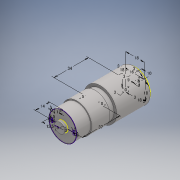
# Autodesk Inventor part: モーター100：1
Saved by Autodesk Inventor 2018 (Build 220112000, 112)
## iProperties
Part Number: モーター100：1
Material: 一般
Document SubType Name: Modeling
Designer: eieio
Density: 1 g/cm^3
Appearance: 溶接 - 軟鋼
Author: eieio
Autodesk Inventor part; units mm, degrees
ref_plane "YZ Plane" through (0, 0, 0) normal (1, 0, 0) x (0, 1, 0)
ref_plane "XZ Plane" through (0, 0, 0) normal (0, 1, 0) x (-1, 0, 0)
ref_plane "XY Plane" through (0, 0, 0) normal (0, 0, 1) x (1, 0, 0)
sketch "スケッチ1" plane through (0, 0, 0) normal (0, 0, 1) x (1, 0, 0)
  line L0 (0, 0) -> (-16, 0)
  line L1 (-16, 0) -> (-16, 34)
  line L2 (-16, 34) -> (0, 34)
  line L3 (0, 34) -> (0, 0)
  line L4 (0, 34) -> (-10, 34)
  line L5 (-10, 34) -> (-10, 37)
  line L6 (-10, 37) -> (0, 37)
  line L7 (0, 37) -> (0, 34)
  line L8 (0, 37) -> (-5, 37)
  line L9 (-5, 34) -> (0, 34)
  line L10 (0, 34) -> (0, 37)
  line L11 (-3, 37) -> (-3, 34)
  line L12 (-13.5, 0) -> (0, 0)
  line L13 (0, 0) -> (0, -37)
  line L14 (0, -37) -> (-13.5, -37)
  line L15 (-13.5, -37) -> (-13.5, 0)
  line L16 (-13.5, 0) -> (-14.5, 0)
  line L17 (-13.5, -23) -> (-13.5, 0)
  line L18 (-13.5, -5) -> (-14.5, -5)
  line L19 (-14.5, -5) -> (-14.5, -23)
  line L20 (-14.5, -23) -> (-13.5, -23)
  line L21 (-13.5, -23) -> (-13.5, -5)
  line L22 (0, -37) -> (-5, -37)
  line L23 (-5, -37) -> (-5, -40)
  line L24 (-5, -40) -> (0, -40)
  line L25 (0, -40) -> (0, -37)
  dimension "d0" = 16
  dimension "d1" = 34
  dimension "d2" = 10
  dimension "d4" = 3
  dimension "d5" = 3
  dimension "d6" = 13.5
  dimension "d7" = 0
  dimension "d10" = 37
  dimension "d11" = 5
  dimension "d12" = 14
  dimension "d13" = 1
  dimension "d14" = 3
  dimension "d15" = 5
  constraints: 52 end point, 11 parallel, 7 horizontal, 6 perpendicular, 4 point on line, 1 midpoint
  measures "d0" distance between parallel lines of L3 L1
  measures "d1" distance between parallel lines of L0 L2
  measures "d2" distance between parallel lines of L7 L5
  measures "d4" distance between parallel lines of L7 L11
  measures "d5" distance between parallel lines of L2 L6
  measures "d6" distance between parallel lines of L13 L15
  measures "d7" distance between parallel lines of L3 L13
  measures "d10" distance between parallel lines of L12 L14
  measures "d11" distance from line of L16.end L18
  measures "d12" distance from line of L20.end L14
  measures "d13" distance between parallel lines of L17 L19
  measures "d14" distance between parallel lines of L22 L24
  measures "d15" distance between parallel lines of L25 L23
revolve "回転1" add sketch "スケッチ1" angle 360 about axis through (0, 34, 0) along (0, -1, 0) contours L13 L14 L15 L0 | L0 L1 L2 L3 | L25 L24 L23 L14 | L15 L20 L19 L18 | L2 L5 L6 L11
chamfer "面取り1" distance 1 angle 45 1 edges at (16, 34, 0)
sketch "スケッチ2" plane through (0, -37, 0) normal (0, -1, 0) x (1, 0, 0)
  circle A0 centre (0, 0) radius 5 projected
  circle A1 centre (0, 0) radius 13.4
  circle A2 centre (0, 0) radius 13.5
  circle A3 centre (0, 0) radius 13.5 projected
  line L0 (-9.9, -2) -> (-11.4, -2)
  line L1 (-11.4, -2) -> (-11.4, 2)
  line L2 (-11.4, 2) -> (-9.9, 2)
  line L3 (-9.9, 2) -> (-9.9, -2)
  line L4 (-9.9, -2) -> (-11.4, 2) construction
  line L5 (-11.4, -2) -> (-9.9, 2) construction
  line L6 (11.4, -2) -> (9.9, -2)
  line L7 (9.9, -2) -> (9.9, 2)
  line L8 (9.9, 2) -> (11.4, 2)
  line L9 (11.4, 2) -> (11.4, -2)
  line L10 (11.4, -2) -> (9.9, 2) construction
  line L11 (9.9, -2) -> (11.4, 2) construction
  line L12 (-13.4, 0) -> (0, 0)
  line L13 (0, 0) -> (13.4, 0)
  point P0 (-10.65, 0)
  point P1 (10.65, 0)
  dimension "d21" = 0
  dimension "d22" = 0.1
  dimension "d23" = 1.5
  dimension "d24" = 1.5
  dimension "d25" = 4
  dimension "d26" = 4
  dimension "d27" = 0
  dimension "d28" = 2
  dimension "d29" = 2
  constraints: 28 end point, 4 midpoint, 4 parallel, 3 horizontal, 2 centre point, 2 coincident, 2 perpendicular, 2 point on circle, 2 point on line
  measures "d21" radial gap between concentric circles of A3 A2
  measures "d22" radial gap between concentric circles of A1 A2
  measures "d23" distance between parallel lines of L3 L1
  measures "d24" distance between parallel lines of L9 L7
  measures "d25" distance between parallel lines of L2 L0
  measures "d26" distance between parallel lines of L6 L8
  measures "d27" distance from line of L12 point (-10.65, 0)
  measures "d28" distance from line of L12.start L1
  measures "d29" distance edge to line of A1 L9
extrude "押し出し1" add sketch "スケッチ2" along normal blind 0.3
extrude "押し出し2" cut sketch "スケッチ2" against normal blind 1 contours L13 L9 L6 L7 | L7 L8 L9 L13 | L12 L1 L2 L3 | L3 L0 L1 L12
sketch "スケッチ3" plane through (0, 34, 0) normal (0, 1, 0) x (1, 0, 0)
  circle A0 centre (0, 0) radius 15 projected
  circle A1 centre (-9, -9) radius 1.5
  circle A2 centre (-9, 9) radius 1.5
  circle A3 centre (9, 9) radius 1.5
  circle A4 centre (9, -9) radius 1.5
  line L0 (9, -9) -> (-9, -9)
  line L1 (-9, -9) -> (-9, 9)
  point P0 (0, 0)
  dimension "d54" = 18
  dimension "d55" = 18
  dimension "d56" = 18
  dimension "d57" = 18
  dimension "d58" = 0
  dimension "d59" = 3
  dimension "d60" = 3
  dimension "d61" = 3
  dimension "d62" = 3
  dimension "d63" = 9
  dimension "d64" = 9
  constraints: 4 centre point, 4 end point, 1 horizontal
  measures "d54" distance of L0.start L0.end
  measures "d55" distance of L1.end L0.end
  measures "d56" distance of A3.centre L1.end
  measures "d57" distance of A3.centre L0.start
  measures "d58" horizontal distance of L1.end L0.end
  measures "d59" diameter of A4
  measures "d60" diameter of A3
  measures "d61" diameter of A2
  measures "d62" diameter of A1
  measures "d63" distance from line of L0 point (0, 0)
  measures "d64" distance from line of L1 point (0, 0)
extrude "押し出し5" cut sketch "スケッチ3" against normal blind 9.5 contours L0 L1 A1 | A1 L1 L0 | A2 | A3 | A4
sketch "スケッチ6" plane through (0, 37, 0) normal (0, 1, 0) x (1, 0, 0)
  circle A0 centre (0, 0) radius 10 projected
  line L0 (-4.3589, -9) -> (4.3589, -9)
  line L1 (-4.3589, 9) -> (4.3589, 9)
  line L2 (0, 10) -> (0, 9)
  line L3 (0, -9) -> (0, -10)
  arc A1 (-4.3589, -9) -> (4.3589, -9) centre (0, 0) ccw
  arc A2 (4.3589, 9) -> (-4.3589, 9) centre (0, 0) ccw
  point P0 (0, 0)
  dimension "d67" = 1
  dimension "d68" = 1
  constraints: 10 point on circle, 8 end point, 2 centre point, 2 coincident, 2 midpoint, 1 horizontal, 1 parallel, 1 point on line
  measures "d67" distance of L3.start L3.end
  measures "d68" distance of L2.start L2.end
extrude "押し出し6" cut sketch "スケッチ6" against normal blind 3 contours L1 L2 A0 | A0 L3 L0 | L2 L1 A0 | A0 L0 L3
